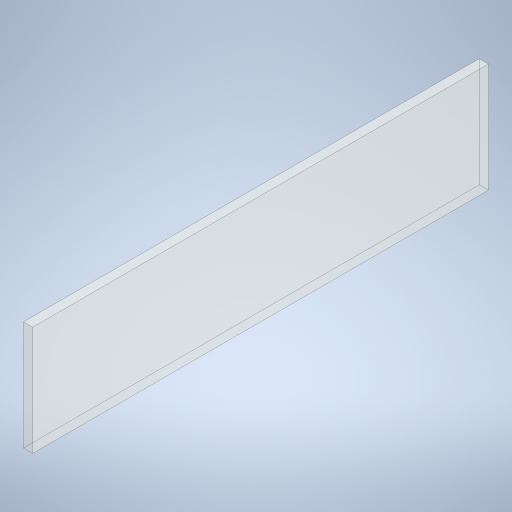
# Autodesk Inventor part: Acrylic Top
Saved by Autodesk Inventor 2024 (Build 280153000, 153)
## iProperties
Created: 2023-07-19
Part Number: Acrylic Top
Material: Acetal Resin, White
Document SubType Name: Modeling
Designer: javie
Density: 1.425 g/cm^3
Appearance: Clear
Author: javie
Autodesk Inventor part; units mm, degrees
ref_plane "YZ Plane" through (0, 0, 0) normal (1, 0, 0) x (0, 1, 0)
ref_plane "XZ Plane" through (0, 0, 0) normal (0, 1, 0) x (-1, 0, 0)
ref_plane "XY Plane" through (0, 0, 0) normal (0, 0, 1) x (1, 0, 0)
sketch "Sketch3" plane through (0, 0, 0) normal (1, 0, 0) x (0, 1, 0)
  line L0 (-23.5, 98) -> (23.5, 98)
  line L1 (23.5, 98) -> (23.5, -98)
  line L2 (23.5, -98) -> (-23.5, -98)
  line L3 (-23.5, -98) -> (-23.5, 98)
  line L4 (-23.5, 98) -> (23.5, -98) construction
  line L5 (23.5, 98) -> (-23.5, -98) construction
  point P0 (0, 0)
  dimension "d8" = 47
  dimension "d9" = 196
  constraints: 12 end point, 2 midpoint, 2 parallel, 1 horizontal, 1 perpendicular
  measures "d8" distance of L1.end L2.end
  measures "d9" distance of L0.end L1.end
extrude "Extrusion3" add sketch "Sketch3" along normal blind 4
body "Solid2"
